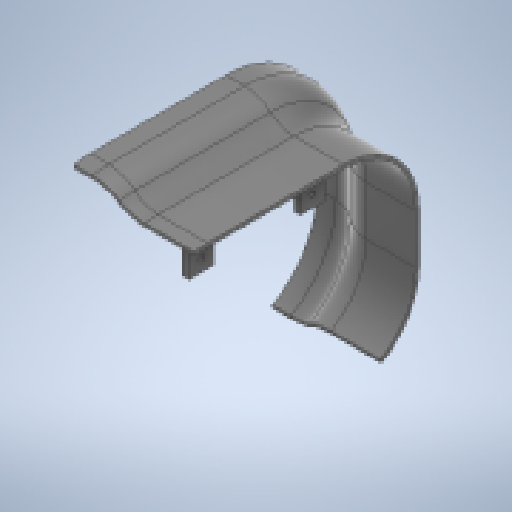
# Autodesk Inventor part: gripper_case_upper2
Saved by Autodesk Inventor 2026.2 (Build 302298010, 298A)
## iProperties
Created: 2026-05-21
Part Number: gripper_case_upper2
Material: ABS Plastic
Document SubType Name: Modeling
Designer: chris
Density: 1.06 g/cm^3
Appearance: Smooth - White
Author: chris
Autodesk Inventor part; units mm, degrees
ref_plane "XY Plane" through (0, 0, 0) normal (0, 0, 1) x (1, 0, 0)
sketch "Sketch2" plane through (0, 0, 0) normal (0, 0, 1) x (1, 0, 0)
  line L0 (0, 0) -> (15, 0)
  arc A0 (35, -7.6393) -> (15, 0) centre (15, -30) ccw
  arc A1 (35, -7.6393) -> (55, -15.2786) centre (55, 14.7214) ccw
  line L1 (55, -15.2786) -> (95, -15.2786)
  dimension "d3" = 15
  dimension "d4" = 30
  dimension "d6" = 20
  dimension "d7" = 30
  dimension "d8" = 40
  constraints: 4 end point, 4 point on circle, 3 tangent, 2 centre point, 2 horizontal
  measures "d3" distance of L0.start L0.end
  measures "d4" distance from line of A0.centre L0
  measures "d6" horizontal distance of A0.centre A0.start
  measures "d7" radius of A1
  measures "d8" distance of L1.start L1.end
sketch "Sketch3" plane through (0, 0, 0) normal (1, 0, 0) x (0, 1, 0)
  line L0 (-1.5, -55) -> (1.5, -55)
  line L1 (1.5, -55) -> (1.5, 55)
  line L2 (1.5, 55) -> (-1.5, 55)
  line L3 (-1.5, 55) -> (-1.5, -55)
  line L4 (-1.5, -55) -> (1.5, 55) construction
  line L5 (1.5, -55) -> (-1.5, 55) construction
  point P0 (0, 0)
  dimension "d9" = 3
  dimension "d10" = 110
  constraints: 12 end point, 2 midpoint, 2 parallel, 1 horizontal, 1 perpendicular
  measures "d9" distance of L2.end L1.end
  measures "d10" distance of L1.end L0.end
sweep "Sweep1" add profiles "Sketch3" path "Sketch2"
sketch "Sketch4" plane through (55, -16.7786, -55) normal (0, -1, 0) x (1, 0, 0)
  line L0 (20, 110) -> (25, 110)
  line L1 (25, 110) -> (25, 90)
  line L2 (25, 90) -> (20, 90)
  line L3 (20, 90) -> (20, 110)
  line L4 (20, 20) -> (25, 20)
  line L5 (25, 20) -> (25, 0)
  line L6 (25, 0) -> (20, 0)
  line L7 (20, 0) -> (20, 20)
  line L8 (0, 110) -> (40, 110) projected
  line L9 (0, 0) -> (40, 0) projected
  line L10 (40, 110) -> (40, 0) projected
  point P0 (-55, 55)
  dimension "d13" = 5
  dimension "d14" = 5
  dimension "d15" = 20
  dimension "d16" = 20
  dimension "d17" = 20
  constraints: 16 end point, 4 parallel, 2 collinear, 2 horizontal, 2 perpendicular, 1 point on line
  measures "d13" distance of L1.end L2.end
  measures "d14" distance of L4.start L4.end
  measures "d15" distance of L4.end L5.end
  measures "d16" distance of L0.end L1.end
  measures "d17" distance between parallel lines of L10 L7
extrude "Extrusion1" add sketch "Sketch4" along normal blind 30
sketch "Sketch5" plane through (80, -16.7786, -35) normal (1, 0, 0) x (0, 0, -1)
  circle A0 centre (10, -20) radius 2.15
  circle A1 centre (-80, -20) radius 2.15
  line L0 (-70, 0) -> (-70, -30) projected
  line L1 (20, 0) -> (20, -30) projected
  line L2 (-90, 0) -> (20, 0) projected
  point P0 (-35, 16.7786)
  dimension "d20" = 4.3
  dimension "d21" = 4.3
  dimension "d22" = 10
  dimension "d23" = 10
  dimension "d24" = 20
  constraints: 2 centre point, 1 horizontal alignment
  measures "d20" diameter of A0
  measures "d21" diameter of A1
  measures "d22" distance from line of L0 A1.centre
  measures "d23" distance from line of L1 A0.centre
  measures "d24" distance from line of L2 A0.centre
extrude "Extrusion2" cut sketch "Sketch5" against normal blind 30
sketch "Sketch6" plane through (0, -1.5, 55) normal (0, 0, 1) x (1, 0, 0)
  line L0 (0, 3) -> (0, 0) projected
  line L1 (0, 0) -> (15, 0) projected
  arc A0 (34, -7.2574) -> (15, 0) centre (15, -28.5) ccw projected
  arc A1 (34, -7.2574) -> (55, -15.2786) centre (55, 16.2214) ccw projected
  line L2 (55, -15.2786) -> (75, -15.2786) projected
  line L3 (75, -15.2786) -> (75, -45.2786) projected
  line L4 (80, -45.2786) -> (75, -45.2786) projected
  line L5 (80, -15.2786) -> (80, -45.2786) projected
  line L6 (80, -15.2786) -> (95, -15.2786) projected
  line L7 (95, -12.2786) -> (95, -15.2786) projected
  line L8 (55, -12.2786) -> (95, -12.2786) projected
  arc A2 (36, -5.0213) -> (55, -12.2786) centre (55, 16.2214) ccw projected
  arc A3 (36, -5.0213) -> (15, 3) centre (15, -28.5) ccw projected
  line L9 (0, 3) -> (15, 3) projected
  line L10 (80, -15.2786) -> (75, -15.2786)
  point P0 (0, 1.5)
  constraints: 2 end point, 1 horizontal
ref_plane "Work Plane1" through (80, 0, 0) normal (1, 0, 0) x (0, 1, 0)
sketch "Sketch8" plane through (80, 0, 0) normal (1, 0, 0) x (0, 1, 0)
  line L0 (-13.7786, 55) -> (-16.7786, 55) projected
  line L1 (-16.7786, 55) -> (-46.7786, 55) projected
  line L2 (-6.5213, 55) -> (-13.7786, 55) projected
  line L3 (-6.5213, 55) -> (1.5, 55) projected
  arc A0 (-15.2786, 55) -> (-75.2786, 115) centre (-75.2786, 55) ccw
  line L4 (-75.2786, 115) -> (-115.2786, 115)
  arc A1 (-115.2786, 115) -> (-167.2402, 85) centre (-115.2786, 55) ccw
  point P0 (0, 0)
  point P1 (-15.2786, 55)
  dimension "d28" = 120
  dimension "d32" = 40
  dimension "d34" = 40
  dimension "d35" = 60
  constraints: 5 point on circle, 2 centre point, 2 end point, 2 point on line, 2 tangent, 1 horizontal, 1 horizontal alignment, 1 midpoint
  measures "d28" diameter of A0
  measures "d32" distance of L4.start L4.end
  measures "d34" distance of A0.centre A1.centre
sweep "Sweep2" add profiles "Sketch6" path "Sketch8" path curves A0 L4 A1 contours L9 A3 A2 L8 L7 L6 L10 L2 A1 A0 L1 L0
fillet "Fillet1" radius 1 8 edges at (7.5, -181.7709, 93.3893) (44.8306, -170.1639, 86.688) (75, -168.5392, 85.75) (26.2399, -179.9751, 92.3525) (75, -165.9411, 84.25) (25.1694, -177.5481, 90.9513) (7.5, -179.1728, 91.8893) (43.7601, -167.7369, 85.2868)
ref_plane "Work Plane2" through (0, -100, 0) normal (0, 1, 0) x (-1, 0, 0)
fillet "Fillet3" radius 5 4 edges at (75, -16.7786, 45) (80, -16.7786, 45) (75, -16.7786, -45) (80, -16.7786, -45)
mirror "Mirror1" about plane through (0, 0, 0) normal (0, 0, 1) of "Sweep2", "Fillet1"
sketch "Sketch16" plane through (0, 1.5, 55) normal (0, 1, 0) x (1, 0, 0)
  line L0 (55, 0) -> (95, 0) projected
  line L1 (0, -76.7786) -> (0, 0) projected
  line L2 (95, 0) -> (0, 0)
  line L3 (0, 0) -> (0, -76.7786)
  line L4 (0, -76.7786) -> (95, -76.7786)
  line L5 (95, -76.7786) -> (95, 0)
  point P0 (0, 55)
  constraints: 8 end point, 2 parallel, 1 horizontal, 1 perpendicular
extrude "Extrusion3" cut sketch "Sketch16" against normal through all
sketch "Sketch17" plane through (80, 0, 0) normal (1, 0, 0) x (0, 1, 0)
  line L0 (-13.7786, 55) -> (-16.7786, 55) projected
  line L1 (-21.7786, 55) -> (-46.7786, 55) projected
  arc A0 (-15.2786, 55) -> (-16.1902, 65.4189) centre (-75.2786, 55) ccw
  line L2 (-75.2786, 55) -> (-16.1902, 65.4189) construction
  line L3 (-75.2786, 55) -> (-15.2786, 55) construction
  point P0 (0, 0)
  dimension "d58" = 10
  dimension "d59" = 60
  constraints: 4 end point, 2 point on circle, 1 centre point, 1 midpoint
  measures "d58" angle of L3 L2
  measures "d59" distance of L2.start L3.end
sketch "Sketch18" plane through (55, -13.7786, 55) normal (0, 0, 1) x (1, 0, 0)
  arc A0 (20, -8) -> (15, -3) centre (15, -8) ccw projected
  line L0 (20, -8) -> (20, -33) projected
  line L1 (25, -33) -> (20, -33) projected
  line L2 (25, -8) -> (25, -33) projected
  arc A1 (30, -3) -> (25, -8) centre (30, -8) ccw projected
  line L3 (30, -3) -> (40, -3) projected
  line L4 (40, 0) -> (40, -3) projected
  line L5 (0, 0) -> (40, 0) projected
  arc A2 (-19, 7.2574) -> (0, 0) centre (0, 28.5) ccw projected
  arc A3 (-19, 7.2574) -> (-40, 15.2786) centre (-40, -16.2214) ccw projected
  line L6 (-55, 15.2786) -> (-40, 15.2786) projected
  line L7 (-55, 12.2786) -> (-55, 15.2786) projected
  line L8 (-55, 12.2786) -> (-40, 12.2786) projected
  arc A4 (-21, 5.0213) -> (-40, 12.2786) centre (-40, -16.2214) ccw projected
  arc A5 (-21, 5.0213) -> (0, -3) centre (0, 28.5) ccw projected
  line L9 (0, -3) -> (15, -3) projected
  line L10 (15, -3) -> (30, -3)
  point P0 (-55, 13.7786)
  constraints: 2 end point, 1 horizontal
sweep "Sweep4" add profiles "Sketch18" path "Sketch17" path curves A0 contours L9 A5 A4 L8 L7 L6 A3 A2 L5 L4 L3 L10
equation "\"d34\" = d32"
body "Solid1"
